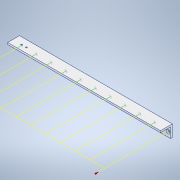
# Autodesk Inventor part: X_Dragchain support
Saved by Autodesk Inventor 2020 (Build 240168000, 168)
## iProperties
Created: 2019-06-04
Part Number: X_Dragchain support
Material: Aluminum 6061
Document SubType Name: Modeling
Designer: LillaHunden
Density: 2.7 g/cm^3
Appearance: Aluminum - Flat
Author: LillaHunden
Autodesk Inventor part; units mm, degrees
ref_plane "YZ Plane" through (0, 0, 0) normal (1, 0, 0) x (0, 1, 0)
ref_plane "XZ Plane" through (0, 0, 0) normal (0, 1, 0) x (-1, 0, 0)
ref_plane "XY Plane" through (0, 0, 0) normal (0, 0, 1) x (1, 0, 0)
sketch "Sketch1" plane through (0, 0, 0) normal (0, 0, 1) x (1, 0, 0)
  line L0 (184.6889, 22.1461) -> (-73.3111, 22.1461)
  line L1 (-73.3111, 22.1461) -> (-73.3111, 42.1461)
  line L2 (-73.3111, 42.1461) -> (184.6889, 42.1461)
  line L3 (184.6889, 42.1461) -> (184.6889, 22.1461)
  point P0 (0, 0)
  dimension "d0" = 258
  dimension "d1" = 20
  constraints: 8 end point, 2 parallel, 1 horizontal, 1 perpendicular
  measures "d0" distance of L1.end L2.end
  measures "d1" distance of L2.end L0.start
extrude "Extrusion1" add sketch "Sketch1" along normal blind 3
sketch "Sketch2" plane through (0, 0, 3) normal (0, 0, 1) x (1, 0, 0)
  line L0 (184.6889, 42.1461) -> (-73.3111, 42.1461) projected
  line L1 (-73.3111, 42.1461) -> (-73.3111, 22.1461) projected
  line L2 (184.6889, 42.1461) -> (-73.3111, 42.1461)
  line L3 (-73.3111, 42.1461) -> (-73.3111, 39.1461)
  line L4 (-73.3111, 39.1461) -> (184.6889, 39.1461)
  line L5 (184.6889, 39.1461) -> (184.6889, 42.1461)
  point P0 (0, 0)
  dimension "d4" = 3
  constraints: 8 end point, 2 parallel, 1 horizontal, 1 perpendicular, 1 point on line
  measures "d4" distance of L3.end L2.end
extrude "Extrusion2" add sketch "Sketch2" along normal blind 17
sketch "Sketch3" plane through (0, 0, 3) normal (0, 0, 1) x (1, 0, 0)
  point P0 (105.6889, 30.1461)
  point P1 (-144.3111, 30.1461)
  point P2 (-119.3111, 30.1461)
  point P3 (-94.3111, 30.1461)
  point P4 (-69.3111, 30.1461)
  point P5 (-44.3111, 30.1461)
  point P6 (-19.3111, 30.1461)
  point P7 (55.6889, 30.1461)
  point P8 (80.6889, 30.1461)
  point P9 (130.6889, 30.1461)
  point P10 (5.6889, 30.1461)
  point P11 (30.6889, 30.1461)
hole "Hole1" at (105.6889, 30.1461, 3) at (-144.3111, 30.1461, 3) at (-119.3111, 30.1461, 3) at (-94.3111, 30.1461, 3) at (-69.3111, 30.1461, 3) at (-44.3111, 30.1461, 3) at (-19.3111, 30.1461, 3) at (55.6889, 30.1461, 3) at (80.6889, 30.1461, 3) at (130.6889, 30.1461, 3) at (5.6889, 30.1461, 3) at (30.6889, 30.1461, 3) direction (0, 0, -1) diameter 3.4 depth 3 countersink diameter 6.3 countersink angle 90
sketch "Sketch4" plane through (-73.3111, 39.1461, 3) normal (0, -1, 0) x (1, 0, 0)
  line L0 (0, 0) -> (0, 17) projected
  point P0 (73.3111, -3)
  point P1 (15, 8.5)
  point P2 (23, 8.5)
  point P3 (0, 8.5)
  dimension "d14" = 8
  dimension "d15" = 15
  constraints: 2 horizontal alignment, 1 midpoint
  measures "d14" distance of point (23, 8.5) point (15, 8.5)
  measures "d15" distance from line of point (15, 8.5) L0
hole "Hole3" at (-58.3111, 39.1461, 11.5) at (-50.3111, 39.1461, 11.5) direction (0, 1, 0) diameter 2.459 depth 8.8 thread size "M3x0.5" class "6H" standard "ISO Metric profile"
sketch "Sketch5" plane through (0, 0, 3) normal (0, 0, 1) x (1, 0, 0)
  point P0 (155.6889, 30.1387)
  point P1 (180.6889, 30.1387)
  point P2 (205.6889, 30.1387)
  point P3 (230.6889, 30.1387)
hole "Hole4" at (155.6889, 30.1387, 3) at (180.6889, 30.1387, 3) at (205.6889, 30.1387, 3) at (230.6889, 30.1387, 3) direction (0, 0, -1) diameter 3.4 depth 3 countersink diameter 6.3 countersink angle 90
body "Solid1"
